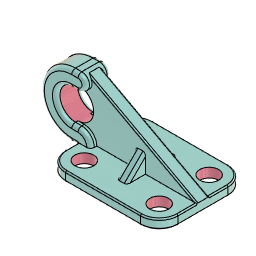
Exercise-21 v1 (Autodesk Fusion 360 design; units mm, degrees)
Autodesk Fusion 360 part; units mm, degrees
note: some values were not read from the file. Chosen so that the rebuilt part matches the saved one: which pieces of a blend or face edit are solid.
sketch "Sketch1" plane through (0, 0, 0) normal (0, 0, 1) x (1, 0, 0)
  line L0 (45, -35) -> (-45, -35)
  line L1 (-45, -35) -> (-45, 35)
  line L2 (-45, 35) -> (45, 35)
  line L3 (45, 35) -> (45, -35)
  line L4 (45, -35) -> (-45, 35) construction
  line L5 (-45, -35) -> (45, 35) construction
  circle A0 centre (30, 20) radius 7.5
  circle A1 centre (-30, 20) radius 7.5
  circle A2 centre (30, -20) radius 7.5
  circle A3 centre (-30, -20) radius 7.5
  dimension "d1" = 90
  dimension "d2" = 70
  dimension "d3" = 15
  dimension "d4" = 15
  dimension "d5" = 15
  dimension "d8" = -60
  dimension "d9" = -40
  constraint horizontal L0
  constraint perpendicular L0 L1
  constraint parallel L0 L2
  constraint parallel L1 L3
  constraint coincident L4 origin
  constraint coincident L5 origin
  measures "d1" distance of L1.end L2.end
  measures "d2" distance of L0.end L1.end
  measures "d3" diameter of A0
  measures "d4" distance of L2 A0.centre
  measures "d5" distance of L3 A0.centre
extrude "Extrude1" add sketch "Sketch1" against normal blind 7.5
fillet "Fillet1" radius 15 4 edges at (-45, -35, -3.75) (-45, 35, -3.75) (45, -35, -3.75) (45, 35, -3.75)
sketch "Sketch2" plane through (0, 0, 0) normal (0, 1, 0) x (1, 0, 0)
  line L0 (45, 7.5) -> (45, 0)
  line L1 (-30, 0) -> (-45, 0)
  line L2 (30, 0) -> (-30, 0)
  line L3 (45, 0) -> (30, 0)
  line L4 (30, 7.5) -> (45, 7.5)
  line L5 (30, 7.5) -> (-30, 7.5)
  line L6 (-45, 7.5) -> (-30, 7.5)
  line L7 (-45, 0) -> (-45, 7.5)
  circle A0 centre (-50, -22.5) radius 12.5
  line L8 (-50, -10) -> (-45, -10)
  line L9 (-50, -35) -> (-45, -35)
  line L10 (-50, -47.5) -> (-45, -47.5)
  line L11 (-50, 2.5) -> (-45, 2.5)
  arc A1 (-50, 2.5) -> (-50, -47.5) centre (-50, -22.5) ccw
  arc A2 (-45, -47.5) -> (-45, -35) centre (-45, -41.25) ccw
  arc A3 (-45.0017, -10) -> (-35, 0) centre (-45, 0) ccw
  line L12 (45, 0) -> (-42.0424, -46.7559)
  dimension "d14" = 25
  dimension "d16" = 30
  dimension "d17" = 5
  dimension "d18" = 5
  dimension "d19" = 5
  dimension "d20" = 5
  constraint coincident A0 L8.start
  constraint tangent A0 L8
  constraint horizontal L8
  constraint coincident A0 L9.start
  constraint horizontal L9
  constraint coincident L1.end L7.start
  constraint tangent L9 A2
  constraint coincident L8 A3.start
  constraint coincident L1 A3.end
  constraint coincident L0.end L3.start
  constraint coincident A2 L12.end
  constraint tangent A2 L12
  measures "d14" diameter of A0
  measures "d16" distance of L6 A0.centre
  measures "d17" horizontal distance of L6.start A0.centre
  measures "d18" distance of L9.start L9.end
  measures "d19" distance of L10.start L10.end
  measures "d20" distance of L11.start L11.end
extrude "Extrude2" add sketch "Sketch2" along normal mid plane 10 contours L1 L2 L3 A0 L8 L9 A2 A3 L12
extrude "Extrude3" add sketch "Sketch2" along normal mid plane 20 contours L1 L7 A0 L8 L9 L10 L11 A1 A2 A3
sketch "Sketch3" plane through (0, 0, 0) normal (1, 0, 0) x (0, 1, 0)
  line L0 (5, 46.7559) -> (5, 0)
  line L1 (20, 0) -> (5, 0)
  line L2 (5, 0) -> (5, 15)
  line L3 (5, 0) -> (20, 0)
  line L4 (20, 0) -> (5, 15)
  line L5 (0, -8) -> (0, 7.5) construction
  line L6 (-20, 0) -> (-5, 15)
  line L7 (-5, 0) -> (-20, 0)
  line L8 (-5, 0) -> (-5, 15)
  dimension "d25" = 15
  dimension "d26" = 15
  constraint coincident L0.end L1.end
  constraint perpendicular L1 L2
  constraint perpendicular L2 L3
  constraint coincident L1.start L3.end
  constraint parallel L0 L5
  constraint symmetric L0.end L5 L7.start
  constraint symmetric L2.end L5 L6.end
  constraint symmetric L1.start L5 L6.start
  measures "d25" distance of L0.end L2.end
  measures "d26" distance of L0.end L1.start
extrude "Extrude4" add sketch "Sketch3" along normal mid plane 8
fillet "Fillet2" radius 3 16 edges at (-37.9295, -10, 7.0717) (-47.5009, -10, 10) (-62.5, -10, 22.5) (-47.5, -10, 35) (-38.75, -10, 41.25) (-47.5, -10, 47.5) (-75, -10, 22.5) (-47.5, -10, -2.5) (-47.5, 10, -2.5) (-75, 10, 22.5) (-47.5, 10, 47.5) (-38.75, 10, 41.25) (-47.5, 10, 35) (-62.5, 10, 22.5) (-47.5009, 10, 10) (-37.9295, 10, 7.0717)
fillet "Fillet3" radius 1 20 edges at (45, -12.5, 0) (40.6066, -30.6066, 0) (0, -35, 0) (-40.6066, -30.6066, 0) (-45, -15, 0) (-45, 15, 0) (-40.6066, 30.6066, 0) (0, 35, 0) (40.6066, 30.6066, 0) (45, 12.5, 0) (1.4788, 5, 23.378) (1.4788, -5, 23.378) (40.6066, -30.6066, -7.5) (0, -35, -7.5) (-40.6066, -30.6066, -7.5) (-45, 0, -7.5) (-40.6066, 30.6066, -7.5) (0, 35, -7.5) (40.6066, 30.6066, -7.5) (45, 0, -7.5)
fillet "Fillet4" radius 2 4 edges at (4, -12.5, 7.5) (-4, -12.5, 7.5) (-4, 12.5, 7.5) (4, 12.5, 7.5)
